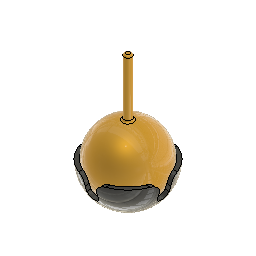
Ball Joint v0 (Autodesk Fusion 360 design; units mm, degrees)
Autodesk Fusion 360 part; units mm, degrees
note: some values were not read from the file. Set by a fixed rule: which sketch regions a step uses.
sketch "Sketch1" plane through (0, 0, 0) normal (0, 1, 0) x (1, 0, 0)
  circle A0 centre (0, 0) radius 50
  circle A1 centre (0, 0) radius 45
  line L0 (0, -85.868) -> (0, 100)
  line L1 (-120, 0) -> (120, 0)
  line L2 (0, 0) -> (5, 0)
  line L3 (5, 0) -> (5, -120)
  line L4 (5, -120) -> (0, -120)
  line L5 (0, -120) -> (0, 0)
  dimension "d1" = 100
  dimension "d2" = 90
  dimension "d3" = 5
  dimension "d4" = 120
  constraint coincident A0.centre A1.centre
  constraint concentric A0 A1
  constraint vertical L0
  constraint perpendicular L0 L1
  constraint horizontal L2
  constraint vertical L3
  constraint horizontal L4
  constraint vertical L5
  measures "d1" diameter of A0
  measures "d2" diameter of A1
  measures "d3" distance of A0.centre L2.end
  measures "d4" distance of A0.centre L4.end
revolve "Revolve1" add sketch "Sketch1" angle 360 about axis through (0, 0, 85.868) along (0, 0, -1) contours A0 A1 L0 L1 picked at (42.8259, 22.1655) makes body 1 in component "Component"
revolve "Revolve1'" add sketch "Sketch1" angle 360 about axis through (0, 0, 120) along (0, 0, -1) separate body contours A0 L0 L3 L4 L5 | A0 A1 L0 L3 L5 | A1 L0 L1 L2 | A1 L1 L3 | A1 L0 L1 L2 L3 L5 makes body 2 in component "Component'"
fillet "Fillet1" radius 2.5 2 edges at (-4.6616, -1.8081, 120) (-4.6616, -1.8081, 44.7214) on bodies 2 in component "Component'"
sketch "Sketch1 (2)" plane through (0, 0, 0) normal (0, 1, 0) x (1, 0, 0) in component "Component"
  line L0 (0, 25) -> (0, 25)
  line L1 (-7.5, 17.5) -> (-7.5, -25)
  line L2 (-7.5, -25) -> (7.5, -25)
  line L3 (7.5, -25) -> (7.5, 17.5)
  line L4 (7.5, 25) -> (-7.5, -25) construction
  line L5 (-7.5, 25) -> (7.5, -25) construction
  arc A0 (0, 25) -> (-7.5, 17.5) centre (0, 17.5) ccw
  arc A1 (7.5, 17.5) -> (0, 25) centre (0, 17.5) ccw
  dimension "d9" = 15
  dimension "d10" = 50
  dimension "d11" = 7.5
  dimension "d12" = 7.5
  constraint parallel L1 L3
  constraint coincident L4 origin
  constraint coincident L5 origin
  constraint coincident L5.start L1
  constraint tangent L1 A0
  constraint coincident L4.start L3
  constraint coincident L4.start L0
  constraint tangent L3 A1
  measures "d9" distance of L1.end L2.end
  measures "d10" distance of L5.start L1.end
  measures "d11" radius of A0
  measures "d12" radius of A1
extrude "Extrude1" cut sketch "Sketch1 (2)" against normal blind 50 bodies 1 in component "Component"
fillet "Fillet1'" radius 10 2 edges at (-7.5, -46.9024, 0) (7.5, -46.9024, 0) on bodies 1 in component "Component"
pattern_circular "C-Pattern1" count 4 over 360 about axis through (0, 0, 1.75) along (0, 0, 1) of "Extrude1", "Fillet1'" in component "Component"
component "Component" placed x (1, 0, 0) y (0, 1, 0) z (0, 0, 1) at (0, 0, 0)
component "Component'" placed x (1, 0, 0) y (0, 1, 0) z (0, 0, 1) at (0, 0, 0)
